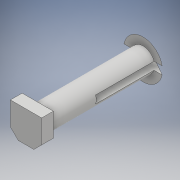
# Autodesk Inventor part: tornillo
Saved by Autodesk Inventor 2018 (Build 220112000, 112)
## iProperties
Created: 2018-04-13
Part Number: tornillo
Material: Genérico
Document SubType Name: Modeling
Designer: se_ma
Density: 1 g/cm^3
Appearance: Valor por defecto
Author: se_ma
Autodesk Inventor part; units mm, degrees
ref_plane "YZ Plane" through (0, 0, 0) normal (1, 0, 0) x (0, 1, 0)
ref_plane "XZ Plane" through (0, 0, 0) normal (0, 1, 0) x (-1, 0, 0)
ref_plane "XY Plane" through (0, 0, 0) normal (0, 0, 1) x (1, 0, 0)
sketch "Boceto1" plane through (0, 0, 0) normal (1, 0, 0) x (0, 1, 0)
  line L0 (0, 0) -> (0, 3)
  line L1 (0, 3) -> (27, 3)
  line L2 (27, 0) -> (0, 0)
  line L3 (27, 0) -> (30, 0)
  line L4 (30, 0) -> (27, 5)
  line L5 (27, 5) -> (27, 3)
  dimension "d0" = 3
  dimension "d1" = 27
  dimension "d2" = 5
  constraints: 12 end point, 2 horizontal, 2 vertical
  measures "d0" distance of L0.start L0.end
  measures "d1" distance of L0.end L1.end
  measures "d2" distance of L2.start L4.end
revolve "Revolución1" add sketch "Boceto1" angle 360 about axis through (0, 27, 0) along (0, -1, 0)
sketch "Boceto2" plane through (0, 0, 0) normal (0, -1, 0) x (1, 0, 0)
  line L0 (0, 0) -> (4, 0)
  line L1 (4, 0) -> (4, 4)
  line L2 (4, 4) -> (-4, 4)
  line L3 (-4, 4) -> (-4, -4)
  line L4 (-4, -4) -> (4, -4)
  line L5 (4, -4) -> (4, 0)
  line L6 (4, -4) -> (4, -2)
  line L7 (4, -4) -> (2, -4)
  line L8 (2, -4) -> (4, -2)
  line L9 (-4, -4) -> (-4, -2)
  line L10 (-4, -4) -> (-2, -4)
  line L11 (-2, -4) -> (-4, -2)
  dimension "d5" = 4
  dimension "d6" = 4
  dimension "d7" = 8
  dimension "d8" = 8
  dimension "d9" = 2
  constraints: 24 end point, 4 perpendicular, 3 point on line, 1 horizontal, 1 midpoint, 1 vertical
  measures "d5" distance of L0.start L0.end
  measures "d6" distance of L0.end L1.end
  measures "d7" distance of L1.end L2.end
  measures "d8" distance of L2.end L3.end
  measures "d9" distance of L3.end L10.end
extrude "Extrusión1" add sketch "Boceto2" along normal blind 3 contours L5 L8 L4 L11 L3 L2 L1
sketch "Boceto4" plane through (0, 0, 0) normal (1, 0, 0) x (0, 1, 0)
  line L0 (30, 0) -> (27, 0)
  line L1 (27, 0) -> (12, 0)
  line L2 (27, -5) -> (27, 5) projected
  line L3 (27, 0) -> (42, 0) construction
  line L4 (12, 0) -> (12, 1)
  line L5 (12, 1) -> (27, 1)
  line L6 (27, 0) -> (27, 1)
  line L7 (12, 0) -> (12, -1)
  line L8 (12, -1) -> (27, -1)
  line L9 (27, -1) -> (27, 0)
  point P0 (0, 0)
  dimension "d15" = 15
  dimension "d16" = 180
  dimension "d17" = 1
  dimension "d18" = 1
  constraints: 18 end point, 6 perpendicular, 3 point on line, 2 horizontal, 1 collinear
  measures "d15" distance of L0.end L1.end
  measures "d16" angle of L1 L3
  measures "d17" distance of L1.end L4.end
  measures "d18" distance of L1.end L7.end
extrude "Extrusión2" cut sketch "Boceto4" along normal mid plane 7
sketch "Boceto5" plane through (0, 27, 0) normal (0, -1, 0) x (1, 0, 0)
  line L0 (-2.8284, -1) -> (2.8284, -1) projected
  line L1 (-2.8284, -1) -> (2.8284, -1)
  arc A0 (2.8284, 1) -> (-2.8284, 1) centre (0, 0) ccw projected
  line L2 (-2.8284, 1) -> (-2.8284, 1)
  line L3 (2.8284, 1) -> (2.8284, -1)
  line L4 (-2.8284, 1) -> (-2.8284, -1)
  line L5 (-2.8284, 1) -> (2.8284, 1) projected
  line L6 (-2.8284, 1) -> (2.8284, 1)
  constraints: 10 end point, 2 perpendicular, 1 collinear, 1 horizontal, 1 vertical
extrude "Extrusión3" cut sketch "Boceto5" against normal blind 7 contours L4 L5 L3 L0
sketch "Boceto6" plane through (-2.8284, 27, 1) normal (1, 0, 0) x (0, 0, -1)
  line L0 (2, 0) -> (0, 0) projected
  line L1 (0, 0) -> (0, 1.2) projected
  line L2 (0, 0) -> (0, 1.2)
  line L3 (0, 1.2) -> (0, 3.2)
  line L4 (0, 0) -> (0, -15) projected
  line L5 (0, 0) -> (2, 0)
  line L6 (2, 0) -> (2, 1.2) projected
  line L7 (2, 0) -> (2, 3.2)
  line L8 (2, 3.2) -> (0, 3.2)
  point P0 (1, -27)
  dimension "d23" = 2
  constraints: 10 end point, 2 perpendicular, 1 collinear, 1 point on line, 1 vertical
  measures "d23" distance of L1.end L3.end
extrude "Extrusión4" cut sketch "Boceto6" along normal mid plane 20
